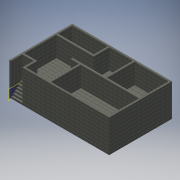
# Autodesk Inventor part: Grundriss_Haus
Saved by Autodesk Inventor 2017 (Build 210142000, 142)
## iProperties
Created: 2017-05-11
Part Number: Grundriss_Haus
Material: Beton, Poren
Document SubType Name: Modeling
Designer: Fake
Density: 1.76203 g/cm^3
Appearance: Flach - Grau 1
Mass: 1.22637e+08 g
Surface Area: 1.748e+06 cm^2
Volume: 6.96e+07 cm^3
Author: Fake
Autodesk Inventor part; units mm, degrees
ref_plane "YZ Plane" through (0, 0, 0) normal (1, 0, 0) x (0, 1, 0)
ref_plane "XZ Plane" through (0, 0, 0) normal (0, 1, 0) x (-1, 0, 0)
ref_plane "XY Plane" through (0, 0, 0) normal (0, 0, 1) x (1, 0, 0)
sketch "Skizze1" plane through (0, 0, 0) normal (0, 0, 1) x (1, 0, 0)
  line L0 (-5680, 3575) -> (5680, 3575)
  line L1 (5680, 3575) -> (5680, -3575)
  line L2 (5680, -3575) -> (-5680, -3575)
  line L3 (-5680, -3575) -> (-5680, 3575)
  line L4 (-7952, 0) -> (7952, 0) projected
  line L5 (0, -5005) -> (0, 5005) projected
  dimension "d0" = 11360
  dimension "d1" = 7150
  constraints: 8 end point, 2 parallel, 1 horizontal, 1 perpendicular, 2 other
  measures "d0" distance of L0.start L0.end
  measures "d1" distance of L2.end L0.start
extrude "Extrusion1" add sketch "Skizze1" along normal blind 1400
ref_plane "Arbeitsebene1" through (-5480, -3575, 0) normal (-1, 0, 0) x (0, 0, 1)
sketch "Skizze2" plane through (-5480, -3575, 0) normal (-1, 0, 0) x (0, 0, 1)
  line L0 (0, 7150) -> (0, 0) projected
  line L1 (0, 7150) -> (1400, 7150) projected
  line L2 (1400, 0) -> (1400, 7150) projected
  line L3 (0, 0) -> (1400, 0) projected
  line L4 (0, 0) -> (200, 0)
  line L5 (0, 0) -> (1400, 0) projected
  line L6 (200, 0) -> (200, 200)
  line L7 (200, 200) -> (400, 200)
  line L8 (400, 200) -> (400, 400)
  line L9 (400, 400) -> (600, 400)
  line L10 (600, 400) -> (600, 600)
  line L11 (600, 600) -> (800, 600)
  line L12 (800, 600) -> (800, 800)
  line L13 (800, 800) -> (1000, 800)
  line L14 (1400, 0) -> (1400, 7150) projected
  line L15 (1400, 0) -> (200, 0)
  line L16 (1000, 800) -> (1000, 1000)
  line L17 (1000, 1000) -> (1200, 1000)
  line L18 (1200, 1000) -> (1200, 1200)
  line L19 (1200, 1200) -> (1400, 1200)
  line L20 (1400, 7150) -> (1400, 0) projected
  line L21 (1400, 1200) -> (1400, 0)
  dimension "d5" = 200
  dimension "d6" = 200
  dimension "d7" = 200
  dimension "d8" = 200
  dimension "d9" = 200
  dimension "d10" = 200
  dimension "d11" = 200
  dimension "d12" = 200
  dimension "d15" = 200
  dimension "d16" = 200
  dimension "d17" = 200
  dimension "d18" = 200
  constraints: 30 end point, 9 perpendicular, 3 vertical, 2 collinear, 2 point on line
  measures "d5" distance between parallel lines of L0 L6
  measures "d6" distance of L6.end L7.end
  measures "d7" distance of L8.end L9.end
  measures "d8" distance of L10.end L11.end
  measures "d9" distance of L4.end L6.end
  measures "d10" distance of L7.end L8.end
  measures "d11" distance of L9.end L10.end
  measures "d12" distance of L11.end L12.end
  measures "d15" distance between parallel lines of L12 L16
  measures "d16" distance between parallel lines of L13 L17
  measures "d17" distance between parallel lines of L16 L18
  measures "d18" distance between parallel lines of L17 L19
extrude "Extrusion3" cut sketch "Skizze2" against normal blind 1280 contours L6 L7 L8 L9 L10 L11 L12 L13 L16 L17 L18 L19 L2 L3
sketch "Skizze4" plane through (0, 0, 1400) normal (0, 0, 1) x (1, 0, 0)
  line L0 (-5480, -3575) -> (-5480, -2375) projected
  line L1 (-5480, -2375) -> (-4200, -2375) projected
  line L2 (-4200, -2375) -> (-4200, -3575) projected
  line L3 (-4200, -3575) -> (5680, -3575) projected
  line L4 (5680, -3575) -> (5680, 3575) projected
  line L5 (5680, 3575) -> (-5680, 3575) projected
  line L6 (-5680, 3575) -> (-5680, -3575) projected
  line L7 (-5680, -3575) -> (-5480, -3575) projected
  line L8 (-5680, -3575) -> (-5680, 3575) projected
  line L9 (-5680, -3575) -> (-5680, 3575)
  line L10 (-5680, 3575) -> (5680, 3575) projected
  line L11 (-5680, 3575) -> (5680, 3575)
  line L12 (5680, -3575) -> (-5680, -3575) projected
  line L13 (5680, 3575) -> (5680, -3575)
  line L14 (5680, -3575) -> (-4200, -3575)
  line L15 (-4200, -3575) -> (-4200, -2275)
  line L16 (-4200, -2275) -> (-5480, -2275)
  line L17 (-5480, -3575) -> (-5480, -2375) projected
  line L18 (-5480, -2275) -> (-5480, -3575)
  line L19 (-5480, -3575) -> (-5680, -3575)
  line L20 (-5680, 3575) -> (-5680, -3575)
  line L21 (-5480, -2275) -> (-5480, 3375)
  line L22 (-5480, 3375) -> (5480, 3375)
  line L23 (5480, 3375) -> (5480, -3375)
  line L24 (5480, -3375) -> (-4000, -3375)
  line L25 (-4000, -3375) -> (-4000, -2075)
  line L26 (-4000, -2075) -> (-5480, -2075)
  dimension "d41" = 200
  dimension "d42" = 200
  dimension "d43" = 200
  dimension "d44" = 200
  dimension "d45" = 200
  dimension "d46" = 1300
  constraints: 30 end point, 10 perpendicular, 3 collinear, 2 point on line, 1 vertical
  measures "d41" distance between parallel lines of L12 L24
  measures "d42" distance between parallel lines of L4 L23
  measures "d43" distance between parallel lines of L5 L22
  measures "d44" distance between parallel lines of L25 L2
  measures "d45" distance between parallel lines of L26 L16
  measures "d46" distance between parallel lines of L12 L16
sketch "Skizze5" plane through (0, 0, 1400) normal (0, 0, 1) x (1, 0, 0)
  line L0 (-5480, -2075) -> (-5480, 3375) projected
  line L1 (-5480, 3375) -> (5480, 3375) projected
  line L2 (5480, 3375) -> (5480, -3375) projected
  line L3 (5480, -3375) -> (-4000, -3375) projected
  line L4 (-4000, -3375) -> (-4000, -2075) projected
  line L5 (-4000, -2075) -> (-5480, -2075) projected
  line L6 (-4200, -3575) -> (5680, -3575) projected
  line L7 (5680, -3575) -> (5680, 3575) projected
  line L8 (5680, 3575) -> (-5680, 3575) projected
  line L9 (-5680, 3575) -> (-5680, -3575) projected
  line L10 (-5680, -3575) -> (-5480, -3575) projected
  line L11 (-5480, -3575) -> (-5480, -2275) projected
  line L12 (-5480, -2275) -> (-4200, -2275) projected
  line L13 (-4200, -2275) -> (-4200, -3575) projected
  line L14 (5480, 3375) -> (5480, -3375) projected
  line L15 (-1140, -3375) -> (-1140, 25)
  line L16 (-1140, 25) -> (5480, 25)
  line L17 (-1340, -3375) -> (-1340, 25)
  line L18 (-1340, 25) -> (-2310, 25)
  line L19 (-2310, 25) -> (-2310, 225)
  line L20 (-2310, 225) -> (5480, 225)
  line L21 (-5480, 1775) -> (-1430, 1775)
  line L22 (-1430, 1775) -> (-1430, 3375)
  line L23 (-5480, 1575) -> (-1230, 1575)
  line L24 (-1230, 1575) -> (-1230, 3375)
  line L25 (-5480, 1575) -> (-5480, 1775)
  line L26 (-1430, 3375) -> (-1230, 3375)
  line L27 (-1330, -3375) -> (-1140, -3375)
  line L28 (5480, 225) -> (5480, 25)
  line L29 (5680, 3575) -> (5680, -3575) projected
  line L30 (5480, 3375) -> (-5480, 3375) projected
  line L31 (1630, 3375) -> (1630, 225)
  line L32 (1430, 3375) -> (1430, 225)
  line L33 (1430, 3375) -> (1630, 3375)
  dimension "d49" = 200
  dimension "d50" = 200
  dimension "d51" = 6620
  dimension "d52" = 3400
  dimension "d53" = 970
  dimension "d54" = 1600
  dimension "d55" = 200
  dimension "d56" = 4050
  dimension "d57" = 200
  dimension "d60" = 3850
  dimension "d61" = 200
  constraints: 34 end point, 13 point on line, 8 perpendicular, 5 collinear, 2 horizontal, 2 vertical, 1 parallel
  measures "d49" distance between parallel lines of L20 L16
  measures "d50" distance between parallel lines of L15 L17
  measures "d51" distance between parallel lines of L2 L15
  measures "d52" distance of L15.start L15.end
  measures "d53" distance of L17.end L18.end
  measures "d54" distance between parallel lines of L1 L21
  measures "d55" distance between parallel lines of L21 L23
  measures "d56" distance between parallel lines of L22 L0
  measures "d57" distance between parallel lines of L24 L22
  measures "d60" distance between parallel lines of L2 L31
  measures "d61" distance between parallel lines of L32 L31
equation "\"d6\" = d5"
equation "\"d7\" = d5"
equation "\"d8\" = d5"
equation "\"d10\" = d9"
equation "\"d11\" = d9"
equation "\"d12\" = d9"
equation "\"d15\" = d6"
equation "\"d16\" = d9"
equation "\"d17\" = d9"
equation "\"d18\" = d9"
